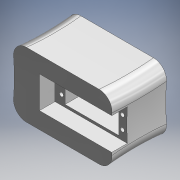
# Autodesk Inventor part: AA048
Saved by Autodesk Inventor 2017 SP1 (Build 210196100, 196)
## iProperties
Created: 2018-01-29
Part Number: AA048
Material: ABS Plastic
Document SubType Name: Modeling
Designer: Zach
Density: 1.06 g/cm^3
Appearance: CR White
Author: Zach
Autodesk Inventor part; units mm, degrees
ref_plane "YZ Plane" through (0, 0, 0) normal (1, 0, 0) x (0, 1, 0)
ref_plane "XZ Plane" through (0, 0, 0) normal (0, 1, 0) x (-1, 0, 0)
ref_plane "XY Plane" through (0, 0, 0) normal (0, 0, 1) x (1, 0, 0)
sketch "Sketch1" plane through (0, 0, 0) normal (0, 0, 1) x (1, 0, 0)
  circle A0 centre (0, 0) radius 1.5
  circle A1 centre (47, 0) radius 1.5
  line L0 (1.5, 0) -> (45.5, 0) construction
  circle A2 centre (0, 10) radius 1.5
  circle A3 centre (47, 10) radius 1.5
  line L1 (1.5, 10) -> (45.5, 10) construction
  line L2 (0, 1.5) -> (0, 8.5) construction
  line L3 (47, 1.5) -> (47, 8.5) construction
  line L4 (-5, 30) -> (52, 30)
  line L5 (52, 30) -> (52, -20)
  line L6 (52, -20) -> (-5, -20)
  line L7 (-5, -20) -> (-5, 30)
  line L8 (2.75, 15.25) -> (44.25, 15.25)
  line L9 (44.25, 15.25) -> (44.25, -5.25)
  line L10 (44.25, -5.25) -> (2.75, -5.25)
  line L11 (2.75, -5.25) -> (2.75, 15.25)
  point P0 (23.5, 15.25)
  point P1 (23.5, 30)
  point P2 (44.25, 5)
  point P3 (52, 5)
  point P4 (2.75, 5)
  point P5 (-5, 5)
  point P6 (0, 5)
  dimension "d0" = 3
  dimension "d1" = 3
  dimension "d2" = 44
  dimension "d3" = 3
  dimension "d4" = 3
  dimension "d6" = 7
  dimension "d7" = 5
  dimension "d8" = 5
  dimension "d11" = 20.5
  dimension "d12" = 41.5
  dimension "d22" = 50
  constraints: 24 end point, 8 point on circle, 7 horizontal alignment, 7 midpoint, 5 vertical alignment, 4 centre point, 4 horizontal, 4 parallel, 2 perpendicular, 2 vertical, 1 coincident
  measures "d0" diameter of A0
  measures "d1" diameter of A1
  measures "d2" distance of L0.start L0.end
  measures "d3" diameter of A2
  measures "d4" diameter of A3
  measures "d6" distance of L3.start L3.end
  measures "d7" distance between parallel lines of L7 L2
  measures "d8" distance between parallel lines of L5 L3
  measures "d11" distance of L8.end L9.end
  measures "d12" distance of L8.start L8.end
  measures "d22" distance of L6.end L4.start
extrude "Extrusion1" add sketch "Sketch1" against normal blind 28
sketch "Sketch2" plane through (0, 0, 0) normal (0, 0, 1) x (1, 0, 0)
  line L0 (-5, 30) -> (52, 30) projected
  line L1 (-5, 30) -> (-26, 30)
  line L2 (-26, 30) -> (-26, -20)
  line L3 (-26, -20) -> (-5, -20)
  line L4 (-5, -20) -> (-5, 30)
  line L5 (2.75, -5.25) -> (2.75, 15.25) projected
  point P0 (0, 0)
  dimension "d15" = 28.75
  constraints: 8 end point, 2 parallel, 1 coincident, 1 horizontal, 1 perpendicular
  measures "d15" distance between parallel lines of L2 L5
extrude "Extrusion2" add sketch "Sketch2" against normal blind 28
sketch "Sketch3" plane through (0, 0, -28) normal (0, 0, -1) x (-1, 0, 0)
  line L0 (-2.75, 15.25) -> (-2.75, -5.25) construction
  line L1 (-2.75, -5.25) -> (-44.25, -5.25) construction
  line L2 (-44.25, -5.25) -> (-44.25, 15.25) construction
  line L3 (-44.25, 15.25) -> (-2.75, 15.25) construction
  circle A0 centre (-47, 10) radius 1.5 construction
  circle A1 centre (0, 10) radius 1.5 construction
  circle A2 centre (-47, 0) radius 1.5 construction
  circle A3 centre (0, 0) radius 1.5 construction
  line L4 (26, 30) -> (-52, 30) projected
  line L5 (-52, 30) -> (-52, -20) projected
  line L6 (-52, -20) -> (26, -20) projected
  line L7 (26, -20) -> (26, 30) projected
extrude "Extrusion3" add sketch "Sketch3" along normal blind 2
sketch "Sketch5" plane through (0, 0, -30) normal (0, 0, -1) x (-1, 0, 0)
  line L0 (-1, -10) -> (-25, -10) construction
  line L1 (-25, -10) -> (-25, 20) construction
  line L2 (-25, 20) -> (-1, 20) construction
  line L3 (-1, 20) -> (-1, -10) construction
  circle A0 centre (-1, -10) radius 1.5
  circle A1 centre (-25, -10) radius 1.5
  circle A2 centre (-25, 20) radius 1.5
  circle A3 centre (-1, 20) radius 1.5
  line L4 (-52, -20) -> (26, -20) projected
  line L5 (26, -20) -> (26, 30) projected
  point P0 (0, 0)
  point P1 (-13, -10)
  point P2 (-1, 5)
  point P3 (26, 5)
  point P4 (-13, -20)
  dimension "d23" = 24
  dimension "d24" = 30
  dimension "d25" = 3
  dimension "d26" = 3
  dimension "d27" = 3
  dimension "d28" = 3
  constraints: 8 end point, 4 centre point, 4 midpoint, 3 coincident, 2 parallel, 1 horizontal, 1 horizontal alignment, 1 perpendicular, 1 vertical alignment
  measures "d23" distance of L1.end L2.end
  measures "d24" distance of L0.end L1.end
  measures "d25" diameter of A0
  measures "d26" diameter of A1
  measures "d27" diameter of A2
  measures "d28" diameter of A3
extrude "Extrusion4" cut sketch "Sketch5" against normal blind 20
sketch "Sketch6" plane through (0, 0, 0) normal (0, 0, 1) x (1, 0, 0)
  line L0 (2.75, -5.25) -> (2.75, 15.25) projected
  line L1 (2.75, 15.25) -> (44.25, 15.25) projected
  line L2 (44.25, 15.25) -> (44.25, -5.25) projected
  line L3 (44.25, -5.25) -> (2.75, -5.25) projected
  circle A0 centre (47, 10) radius 1.5 projected
  circle A1 centre (0, 10) radius 1.5 projected
  circle A2 centre (47, 0) radius 1.5 projected
  circle A3 centre (0, 0) radius 1.5 projected
  line L4 (-26, 30) -> (52, 30) projected
  line L5 (-26, 30) -> (-26, -20) projected
  line L6 (52, -20) -> (-26, -20) projected
  line L7 (52, 30) -> (52, -20) projected
  line L8 (52, 30) -> (52, -20) projected
  line L9 (52, 17.25) -> (-5, 17.25)
  line L10 (-5, 17.25) -> (-5, -7.25)
  line L11 (-5, -7.25) -> (52, -7.25)
  line L12 (52, -7.25) -> (52, 17.25)
  point P0 (44.25, 5)
  point P1 (52, 5)
  dimension "d35" = 7.75
  dimension "d36" = 2
  constraints: 8 end point, 2 midpoint, 2 parallel, 1 horizontal, 1 horizontal alignment, 1 perpendicular, 1 point on line
  measures "d35" distance between parallel lines of L0 L10
  measures "d36" distance between parallel lines of L9 L1
extrude "Extrusion5" add sketch "Sketch6" along normal blind 12 contours L4 L7 L9 L10 L11 L6 L5
sketch "Sketch7" plane through (-26, -20, -30) normal (-1, 0, 0) x (0, 0, 1)
  line L0 (42, 0) -> (42, 12.75) projected
  line L1 (0, 0) -> (0, 50) projected
  arc A0 (42, 0) -> (0, 0) centre (21, -198.8944) ccw
  line L2 (42, 50) -> (0, 50) projected
  line L3 (42, 37.25) -> (42, 50) projected
  arc A1 (0, 50) -> (42, 50) centre (21, 248.8944) ccw
  line L4 (0, 0) -> (42, 0) projected
  point P0 (30, 20)
  dimension "d39" = 200
  dimension "d40" = 200
  constraints: 4 point on circle, 2 centre point
  measures "d39" radius of A0
  measures "d40" radius of A1
extrude "Extrusion6" cut sketch "Sketch7" against normal through all
sketch "Sketch8" plane through (0, 0, 12) normal (0, 0, 1) x (1, 0, 0)
  line L0 (-26, 30) -> (52, 30) projected
  line L1 (52, -20) -> (-26, -20) projected
  arc A0 (52, 30) -> (52, -20) centre (250.4313, 5) ccw
  arc A1 (-26, -20) -> (-26, 30) centre (-224.4313, 5) ccw
  line L2 (52, -20) -> (52, 30)
  line L3 (-26, 30) -> (-26, -20)
  line L4 (-26, 28.8944) -> (52, 28.8944) projected
  point P0 (0, 0)
  dimension "d43" = 200
  dimension "d44" = 200
  constraints: 4 end point, 4 point on circle, 2 centre point, 1 perpendicular, 1 vertical
  measures "d43" radius of A0
  measures "d44" radius of A1
extrude "Extrusion7" cut sketch "Sketch8" against normal through all contours A1 L4 L3 | L2 L4 A0 | A1 L3 L4 | L4 L2 A0
fillet "Fillet3" radius 10 4 edges at (-25.8638, -18.8944, -9) (-25.8638, 28.8944, -9) (51.8638, -18.8944, -9) (51.8638, 28.8944, -9)
body "Solid1"
